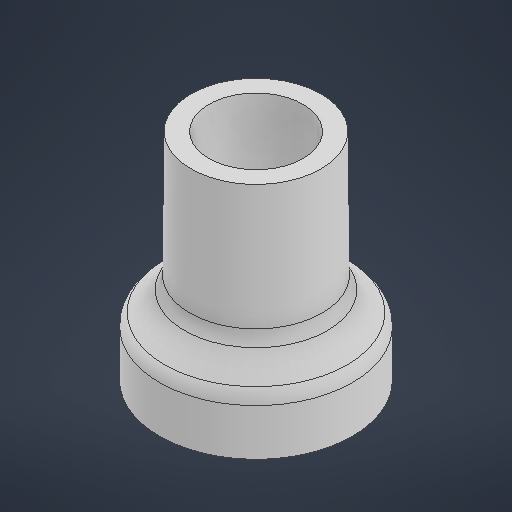
# Autodesk Inventor part: BlowerInletPort
Saved by Autodesk Inventor 2026 (Build 300175050, 175E)
## iProperties
Created: 2025-07-02
Part Number: BlowerInletPort
Material: Generic
Document SubType Name: Modeling
Designer: user
Density: 1 g/cm^3
Appearance: Default
Author: user
## iProperties of the stored document BlowerInletPort_3DPrint.ipt
Created: 2025-07-02
Part Number: BlowerInletPort_3DPrint
Material: Generic
Document SubType Name: Modeling
Designer: user
Density: 1 g/cm^3
Appearance: Default
Author: user
Autodesk Inventor part; units mm, degrees
ref_plane "YZ Plane" through (0, 0, 0) normal (1, 0, 0) x (0, 1, 0)
ref_plane "XZ Plane" through (0, 0, 0) normal (0, 1, 0) x (-1, 0, 0)
ref_plane "XY Plane" through (0, 0, 0) normal (0, 0, 1) x (1, 0, 0)
sketch "Sketch2" plane through (0, 0, 0) normal (0, 0, 1) x (1, 0, 0)
  line L0 (12.85, 9) -> (13.1, 0)
  line L1 (0, 0) -> (13.1, 0) construction
  line L2 (0, 9) -> (12.85, 9) construction
  line L3 (0, 0) -> (0, 9) construction
  line L4 (16.1, 0) -> (16.1, 9)
  line L5 (16.1, 9) -> (11.05, 14.05)
  line L6 (11.05, 14.05) -> (10.85, 36.05)
  line L7 (10.85, 36.05) -> (7.85, 36.05)
  line L8 (7.85, 36.05) -> (7.85, 9)
  line L9 (7.85, 9) -> (12.85, 9)
  line L10 (13.1, 0) -> (16.1, 0)
  line L11 (0, -7.21) -> (0, 43.26) projected
  dimension "d0" = 13.1
  dimension "d1" = 12.85
  dimension "d2" = 9
  dimension "d3" = 3
  dimension "d4" = 45
  dimension "d5" = 11.05
  dimension "d6" = 22
  dimension "d7" = 10.85
  dimension "d8" = 3
  constraints: 22 end point, 5 horizontal, 3 horizontal alignment, 3 vertical, 1 point on line
  measures "d0" distance of L1.start L0.end
  measures "d1" distance of L2.start L0.start
  measures "d2" distance of L1.start L2.start
  measures "d3" distance of L4.start L0.end
  measures "d4" angle of L2 L5
  measures "d5" horizontal distance of L1.start L5.end
  measures "d6" vertical distance of L5.end L6.end
  measures "d7" horizontal distance of L1.start L6.end
  measures "d8" distance from line of L6.end L8
revolve "Revolution1" add sketch "Sketch2" angle 360 about axis through (0, -10, 0) along (0, 1, 0)
fillet "Fillet2" radius 3 2 edges at (-11.05, 14.05, 0) (-16.1, 9, 0)
body "Solid1"
